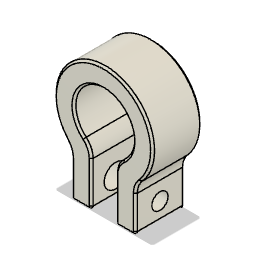
240708 air pipe clamp v2 (Autodesk Fusion 360 design; units mm, degrees)
Autodesk Fusion 360 part; units mm, degrees
sketch "air pipe clamp base" plane through (0, 0, 0) normal (0, 0, 1) x (1, 0, 0)
  line L0 (-6.5, -9.2601) -> (-6.5, -16.5993)
  line L1 (-6.5, -16.5993) -> (-2.5, -16.5993)
  line L2 (2.5, -16.5993) -> (6.5, -16.5993)
  line L3 (6.5, -16.5993) -> (6.5, -9.2601)
  line L4 (-2.5, -16.5993) -> (-2.5, -7.5993)
  line L5 (2.5, -16.5993) -> (2.5, -7.5993)
  arc A0 (7.5, -6.6144) -> (-7.5, -6.6144) centre (0, 0) ccw
  arc A1 (3.9, -4.5596) -> (-3.9, -4.5596) centre (0, 0) ccw
  line L6 (0, 0) -> (0, -19.8599) construction
  arc A2 (-2.5, -7.5993) -> (-3.9, -4.5596) centre (-6.5, -7.5993) ccw
  arc A3 (3.9, -4.5596) -> (2.5, -7.5993) centre (6.5, -7.5993) ccw
  arc A4 (-6.5, -9.2601) -> (-7.5, -6.6144) centre (-10.5, -9.2601) ccw
  arc A5 (7.5, -6.6144) -> (6.5, -9.2601) centre (10.5, -9.2601) ccw
  point P0 (-6.5, -7.5993)
  dimension "d1" = 12
  dimension "d3" = 4
  dimension "d4" = 5
  dimension "d5" = 4
  dimension "d6" = 4
  dimension "d7" = 9
  dimension "d8" = 4
  constraint coincident A0.centre A1.centre
  constraint vertical L0
  constraint perpendicular L0 L1
  constraint perpendicular L0 L2
  constraint perpendicular L2 L3
  constraint perpendicular L1 L4
  constraint perpendicular L2 L5
  constraint vertical L6
  constraint collinear L1 L2
  constraint tangent L4 A2
  constraint tangent A1 A2
  constraint tangent L5 A3
  constraint tangent A1 A3
  constraint equal A2 A3
  constraint coincident P0 L0
  constraint coincident P0 A0
  constraint tangent L0 A4
  constraint tangent A0 A4
  constraint equal A2 A4
  constraint tangent L3 A5
  constraint tangent A0 A5
  constraint equal A2 A5
  measures "d1" diameter of A1
  measures "d3" distance of A0 A1
  measures "d4" distance of L4 L5
  measures "d5" distance of L0 L4
  measures "d6" distance of L3 L5
  measures "d7" distance of P0 L1
  measures "d8" radius of A2
extrude "Extrude1" add sketch "air pipe clamp base" along normal blind 10
sketch "screw holes" plane through (-6.5, 0, 0) normal (-1, 0, 0) x (0, 0, 1)
  line L0 (0, -9.2601) -> (0, -16.5993)
  line L1 (0, -16.5993) -> (10, -16.5993)
  line L2 (10, -16.5993) -> (10, -9.2601)
  line L3 (10, -9.2601) -> (0, -9.2601)
  line L4 (0, -9.2601) -> (10, -16.5993) construction
  line L5 (10, -9.2601) -> (0, -16.5993) construction
  point P0 (5, -12.9297)
  constraint coincident L0.start L3.end
  constraint coincident L1.end L2.start
  constraint coincident L2.end L3.start
  constraint coincident L0.end L1.start
  constraint midpoint L4 P0
hole "Hole1" at (-6.5, -12.9297, 5) direction (1, 0, 0) diameter 4.7 depth 5 tip angle 180
hole "Hole2" at (-6.5, -12.9297, 5) direction (1, 0, 0) diameter 3.3 depth 25 tip angle 180
fillet "Fillet1" radius 0.6 4 edges at (-6.5, -16.5993, 5) (-2.5, -16.5993, 5) (2.5, -16.5993, 5) (6.5, -16.5993, 5)
chamfer "Chamfer1" distance 0.4 angle 45 2 faces at (-3.8333, -10.9529, 10) (-3.8333, -10.9529, 0)
named bodies: "air pipe clamp"
